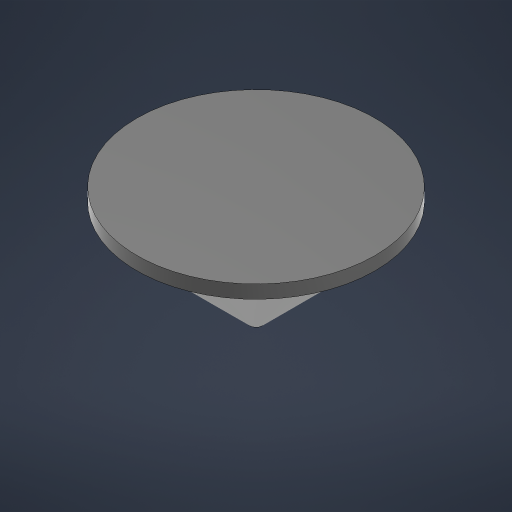
# Autodesk Inventor part: Camera_mirror
Saved by Autodesk Inventor 2024.2 (Build 282272000, 272)
## iProperties
Created: 2023-12-21
Part Number: Camera_mirror
Material: 一般
Document SubType Name: Modeling
Designer: Hanaoka
Density: 1 g/cm^3
Appearance: 既定
Author: Hanaoka
Autodesk Inventor part; units mm, degrees
ref_plane "YZ Plane" through (0, 0, 0) normal (1, 0, 0) x (0, 1, 0)
ref_plane "XZ Plane" through (0, 0, 0) normal (0, 1, 0) x (-1, 0, 0)
ref_plane "XY Plane" through (0, 0, 0) normal (0, 0, 1) x (1, 0, 0)
sketch "スケッチ1" plane through (0, 0, 0) normal (0, 0, 1) x (1, 0, 0)
  line L0 (-25, 25) -> (-1.4142, 1.4142)
  line L1 (1.4142, 1.4142) -> (25, 25)
  line L2 (-25, 25) -> (25, 25)
  line L3 (0, 0) -> (0, 25) construction
  line L4 (-27, 28) -> (27, 28)
  line L5 (27, 28) -> (27, 25)
  line L6 (27, 25) -> (-27, 25)
  line L7 (-27, 25) -> (-27, 28)
  line L8 (0, -5.6) -> (0, 33.6) projected
  line L9 (0, 0) -> (0, 28)
  arc A0 (-1.4142, 1.4142) -> (1.4142, 1.4142) centre (0, 2.8284) ccw
  point P0 (25, 25)
  point P1 (0, 0.8284)
  dimension "d0" = 50
  dimension "d1" = 25
  dimension "d2" = 54
  dimension "d3" = 3
  dimension "d5" = 2
  constraints: 18 end point, 4 point on line, 2 horizontal, 2 midpoint, 2 parallel, 2 perpendicular, 2 point on circle, 2 tangent, 1 centre point, 1 coincident, 1 other
  measures "d0" distance of L0.start L1.end
  measures "d1" distance of L3.start L3.end
  measures "d2" distance of L4.start L4.end
  measures "d3" distance of L6.end L4.start
  measures "d5" radius of A0
revolve "回転1" add sketch "スケッチ1" angle 360 about axis through (0, -10, 0) along (0, 1, 0) contours L8 L4 L5 L6 L2 | L2 L1 A0 L8
